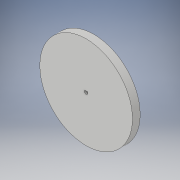
# Autodesk Inventor part: pibot_wheel_1
Saved by Autodesk Inventor 2018.1 (Build 221171000, 171)
## iProperties
Created: 2018-05-04
Part Number: pibot_wheel_1
Material: Generic
Document SubType Name: Sheet Metal
Designer: mmarkle
Density: 1 g/cm^3
Sheet Metal Rule: Default
Appearance: Default
Author: mmarkle
Autodesk Inventor part; units mm, degrees
ref_plane "YZ Plane" through (0, 0, 0) normal (1, 0, 0) x (0, 1, 0)
ref_plane "XZ Plane" through (0, 0, 0) normal (0, 1, 0) x (-1, 0, 0)
ref_plane "XY Plane" through (0, 0, 0) normal (0, 0, 1) x (1, 0, 0)
sketch "Sketch1" plane through (0, 0, 0) normal (0, 0, 1) x (1, 0, 0)
  circle A0 centre (0, 0) radius 38.1
  dimension "d0" = 76.2
  measures "d0" diameter of A0
extrude "Plate1" add sketch "Sketch1" along normal blind 6.35
sketch "Sketch2" plane through (0, 0, 6.35) normal (0, 0, 1) x (1, 0, 0)
  arc A0 (-1.113, 0.9652) -> (1.113, 0.9652) centre (0, 0) ccw
  line L0 (-1.113, 0.9652) -> (1.113, 0.9652)
  arc A1 (1.113, 0.9652) -> (-1.113, 0.9652) centre (0, 0) ccw construction
  dimension "d2" = 2.9464
  dimension "d4" = 2.4384
  constraints: 4 point on circle, 2 centre point, 2 end point, 1 coincident, 1 horizontal
  measures "d2" diameter of A0
extrude "Cut1" cut sketch "Sketch2" against normal blind 6.35
equation "\"d5\" = Thickness"
equation "\"d1\" = Thickness"
equation "\"BendRadius\" = Thickness"
equation "\"BendReliefWidth\" = Thickness"
equation "\"BendReliefDepth\" = 0.5 * Thickness"
equation "\"CornerReliefSize\" = 4 * Thickness"
equation "\"MinimumRemnant\" = 2 * Thickness"
equation "\"TransitionRadius\" = BendRadius"
equation "\"JacobiRadiusSize\" = BendRadius"
equation "\"GapSize\" = Thickness"
equation "\"smallerness\" = 0.0254"
equation "\"Thickness\" = 6.35"
body "Solid1"
